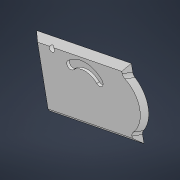
# Autodesk Inventor part: Deo1 with Sketch
Saved by Autodesk Inventor 2022.1 (Build 261234000, 234)
## iProperties
Created: 2021-08-16
Part Number: Deo1 with Sketch
Material: Generic
Document SubType Name: Modeling
Designer: Nedeljko Š.
Density: 1 g/cm^3
Appearance: Default
Author: Nedeljko Š.
Autodesk Inventor part; units mm, degrees
ref_plane "YZ Plane" through (0, 0, 0) normal (1, 0, 0) x (0, 1, 0)
ref_plane "XZ Plane" through (0, 0, 0) normal (0, 1, 0) x (-1, 0, 0)
ref_plane "XY Plane" through (0, 0, 0) normal (0, 0, 1) x (1, 0, 0)
sketch "Sketch1" plane through (0, 0, 0) normal (0, 0, 1) x (1, 0, 0)
  line L0 (-76.521, -76.4496) -> (100, -41.2311)
  line L1 (100, -41.2311) -> (76.521, 76.4496)
  line L2 (76.521, 76.4496) -> (-100, 41.2311)
  line L3 (-100, 41.2311) -> (-76.521, -76.4496)
  line L4 (-76.521, -76.4496) -> (76.521, 76.4496) construction
  line L5 (100, -41.2311) -> (-100, 41.2311) construction
  point P0 (0, 0)
  point P1 (0, 0)
  dimension "d0" = 180
  dimension "d1" = 120
  dimension "d23" = 100
  constraints: 12 end point, 3 midpoint, 2 parallel, 1 perpendicular
  measures "d0" distance of L2.end L1.end
  measures "d1" distance of L1.end L0.end
  measures "d23" horizontal distance of point (0, 0) L2.end
extrude "Extrusion1" add sketch "Sketch1" along normal blind 10 draft -45
sketch "Sketch2" plane through (0, 0, 0) normal (0, 0, 1) x (1, 0, 0)
  circle A0 centre (53.937, 10.7612) radius 55
  line L0 (100, -41.2311) -> (76.521, 76.4496) construction
  line L1 (0, 0) -> (88.2605, 17.6093) construction
  dimension "d0" = 180
  dimension "d4" = 110
  dimension "d5" = 55
  constraints: 2 end point, 1 centre point, 1 midpoint, 1 point on line
  measures "d4" diameter of A0
  measures "d5" distance of A0.centre L1.start
extrude "Extrusion2" add sketch "Sketch2" along normal blind 10 draft -30
fillet "Fillet1" radius 10 2 edges at (75.0191, 58.4193, 5.0006) (91.694, -25.1576, 5.0006)
sketch "Sketch3" plane through (0, 0, 10) normal (0, 0, 1) x (1, 0, 0)
  line L0 (-68.6708, -64.6863) -> (-88.2367, 33.3809) projected
  line L1 (-88.2367, 33.3809) -> (68.6708, 64.6863) projected
  point P0 (0, 0)
  point P1 (-61.4584, 35.8123)
hole "Hole1" at (-61.4584, 35.8123, 10) direction (0, 0, -1) diameter 10 depth 18
sketch "Sketch4" plane through (0, 0, 10) normal (0, 0, 1) x (1, 0, 0)
  arc A0 (26.8701, 26.8701) -> (-26.8701, 26.8701) centre (0, 0) ccw construction
  arc A1 (31.8198, 31.8198) -> (-31.8198, 31.8198) centre (0, 0) ccw
  arc A2 (21.9203, 21.9203) -> (-21.9203, 21.9203) centre (0, 0) ccw
  arc A3 (21.9203, 21.9203) -> (31.8198, 31.8198) centre (26.8701, 26.8701) ccw
  arc A4 (-31.8198, 31.8198) -> (-21.9203, 21.9203) centre (-26.8701, 26.8701) ccw
  dimension "d18" = 90
  dimension "d19" = 7
  dimension "d20" = 38
  constraints: 10 point on circle, 5 centre point, 4 tangent, 1 coincident, 1 horizontal alignment
  measures "d19" radius of A3
  measures "d20" radius of A0
extrude "Extrusion3" cut sketch "Sketch4" against normal blind 5
sketch "Sketch5" plane through (0, 0, 0) normal (0, 0, -1) x (-1, 0, 0)
  arc A0 (-83.5829, 57.0874) -> (-99.091, -20.6413) centre (-53.937, 10.7612) ccw projected
  line L0 (-79.2266, 62.8887) -> (-76.521, 76.4496) projected
  line L1 (-76.521, 76.4496) -> (100, 41.2311) projected
  line L2 (100, 41.2311) -> (76.521, -76.4496) projected
  circle A1 centre (61.4584, 35.8123) radius 5 projected
  line L3 (76.521, -76.4496) -> (-100, -41.2311) projected
  line L4 (-100, -41.2311) -> (-97.2944, -27.6702) projected
  line L5 (-79.2266, 62.8887) -> (-83.5829, 57.0874)
  line L6 (-97.2944, -27.6702) -> (-99.091, -20.6413)
  arc A2 (21.9203, 21.9203) -> (-21.9203, 21.9203) centre (0, 0) ccw projected
  arc A3 (21.9203, 21.9203) -> (31.8198, 31.8198) centre (26.8701, 26.8701) ccw projected
  arc A4 (31.8198, 31.8198) -> (-31.8198, 31.8198) centre (0, 0) ccw projected
  arc A5 (-31.8198, 31.8198) -> (-21.9203, 21.9203) centre (-26.8701, 26.8701) ccw projected
  dimension "d0" = 180
  constraints: 4 end point
body "Solid1"
